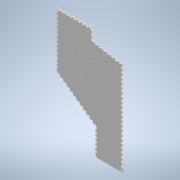
# Autodesk Inventor part: 00_Baseplate_Simmo_base
Saved by Autodesk Inventor 2022 (Build 260153000, 153)
## iProperties
Created: 2022-04-28
Part Number: 00_Baseplate_Simmo_base
Material: Generisch
Document SubType Name: Modeling
Designer: diederichbenedict
Density: 1 g/cm^3
Appearance: Vorgabe
Author: diederichbenedict
Autodesk Inventor part; units mm, degrees
ref_plane "YZ Plane" through (0, 0, 0) normal (1, 0, 0) x (0, 1, 0)
ref_plane "XZ Plane" through (0, 0, 0) normal (0, 1, 0) x (-1, 0, 0)
ref_plane "XY Plane" through (0, 0, 0) normal (0, 0, 1) x (1, 0, 0)
ref_plane "Arbeitsebene1" through (0, 0, 0) normal (0, 0, 1) x (1, 0, 0)
sketch "Skizze1" plane through (0, 0, 0) normal (0, 0, 1) x (1, 0, 0)
  line L0 (91.8818, 443.0401) -> (90.2278, 433.6598) projected
  line L1 (120, 0) -> (126, 0)
  line L2 (126, 0) -> (126, 460)
  line L3 (126, 460) -> (-21.6976, 486.0431)
  line L4 (-21.6976, 538.0431) -> (-196, 538.0431)
  line L5 (-196, 538.0431) -> (-196, 268.0431)
  line L6 (-196, 268.0431) -> (-6, 130)
  line L7 (-6, 130) -> (-6, 0)
  circle A0 centre (58.4, 5) radius 1.4 projected
  line L8 (88.6, 0) -> (31.4, 0) projected
  line L9 (87.5, 10) -> (32.5, 10) projected
  line L10 (120, 0) -> (0, 0)
  line L11 (126, 0) -> (-6, 0)
  line L12 (64.2504, 447.9123) -> (88.7659, 443.5895) construction
  line L13 (-114.6675, 285.8993) -> (-136.5111, 301.7696) construction
  line L14 (-134.4827, 366.1267) -> (-158.3225, 378.8026) construction
  line L15 (-21.6976, 486.0431) -> (-21.6976, 538.0431)
  circle A1 centre (78.4, 5) radius 1.4 projected
  circle A2 centre (38.4, 5) radius 1.4 projected
  circle A3 centre (100.9244, 442.0092) radius 4 construction
  circle A4 centre (31.4122, 427.865) radius 4 construction
  circle A5 centre (96.4095, 416.4042) radius 4 construction
  circle A6 centre (35.927, 453.47) radius 4 construction
  line L16 (51.7328, 440.252) -> (83.0647, 434.7274) construction
  line L17 (83.0647, 434.7274) -> (84.7881, 444.5016) construction
  line L18 (84.7881, 444.5016) -> (53.4563, 450.0262) construction
  line L19 (53.4563, 450.0262) -> (51.7328, 440.252) construction
  line L20 (80.7877, 445.6487) -> (93.6153, 443.3868) construction
  line L21 (93.6153, 443.3868) -> (94.8156, 450.1944) construction
  line L22 (94.8156, 450.1944) -> (106.0791, 448.2083) construction
  arc A7 (108.5126, 444.7329) -> (106.0791, 448.2083) centre (105.5582, 445.2539) ccw construction
  line L23 (108.5126, 444.7329) -> (102.6086, 411.2495) construction
  arc A8 (99.1332, 408.816) -> (102.6086, 411.2495) centre (99.6541, 411.7704) ccw construction
  line L24 (99.1332, 408.816) -> (26.2574, 421.666) construction
  arc A9 (23.8239, 425.1413) -> (26.2574, 421.666) centre (26.7784, 424.6204) ccw construction
  line L25 (23.8239, 425.1413) -> (29.728, 458.6248) construction
  arc A10 (33.2033, 461.0583) -> (29.728, 458.6248) centre (32.6824, 458.1038) ccw construction
  line L26 (33.2033, 461.0583) -> (44.5085, 459.0649) construction
  line L27 (44.5085, 459.0649) -> (43.3082, 452.2573) construction
  line L28 (43.3082, 452.2573) -> (56.1358, 449.9955) construction
  line L29 (56.1358, 449.9955) -> (57.3361, 456.803) construction
  line L30 (57.3361, 456.803) -> (81.988, 452.4562) construction
  line L31 (81.988, 452.4562) -> (80.7877, 445.6487) construction
  line L32 (32.5, 5.1) -> (32.5, 10) projected
  line L33 (87.5, 10) -> (87.5, 5.1) projected
  line L34 (87.5, 5.1) -> (88.6, 5.1) projected
  line L35 (88.6, 5.1) -> (88.6, 0) projected
  line L36 (31.4, 0) -> (31.4, 5.1) projected
  line L37 (31.4, 5.1) -> (32.5, 5.1) projected
  point P0 (126, 5)
  dimension "d1" = 90
  dimension "d66" = 130
  dimension "d69" = 460
  dimension "d70" = 190
  dimension "d71" = 270
  constraints: 20 end point, 3 horizontal, 3 parallel, 1 perpendicular, 1 point on line, 1 vertical
  measures "d1" angle of L5 L4
  measures "d66" vertical distance of L1.start L6.end
  measures "d69" distance of L1.end L2.end
  measures "d70" distance between parallel lines of L5 L7
  measures "d71" distance of L4.end L5.end
extrude "Extrusion1" add sketch "Skizze1" along normal blind 6 contours L10 L35 L34 L33 L9 L32 L37 L36 L11 L7 L6 L5 L4 L15 L3 L2 L1 | L8 L36 L37 L32 L9 L33 L34 L35 | A0 | A1 | A2
sketch "Skizze2" plane through (0, 0, 0) normal (0, 0, -1) x (-1, 0, 0)
  line L0 (-126, 0) -> (-120, 0)
  line L1 (-120, 0) -> (-120, 10)
  line L2 (-120, 10) -> (-126, 10)
  line L3 (-126, 10) -> (-126, 0)
  circle A0 centre (-123, 15) radius 1.5
  point P0 (0, 0)
  dimension "d8" = 6
  dimension "d9" = 10
  dimension "d15" = 3
  dimension "d16" = 5
  constraints: 8 end point, 2 parallel, 2 point on line, 1 centre point, 1 horizontal, 1 perpendicular
  measures "d8" distance of L2.end L1.end
  measures "d9" distance of L1.end L0.end
  measures "d15" diameter of A0
  measures "d16" distance from line of A0.centre L2
extrude "Extrusion2" cut sketch "Skizze2" against normal through all
sketch "Skizze3" plane through (0, 0, 0) normal (0, 0, -1) x (-1, 0, 0)
  line L0 (196, 268.0431) -> (6, 130) projected
  line L1 (196, 538.0431) -> (196, 268.0431) projected
  line L2 (21.6976, 538.0431) -> (196, 538.0431) projected
  line L3 (-126, 460) -> (21.6976, 486.0431) projected
pattern_linear "Rechteckige Anordnung1" count 24 spacing 20 along (0, 1, 0) of "Extrusion2"
sketch "Skizze4" plane through (0, 0, 0) normal (0, 0, -1) x (-1, 0, 0)
  line L0 (-120, 461.058) -> (-110.1519, 462.7944)
  line L1 (-110.1519, 462.7944) -> (-109.11, 456.8856)
  line L2 (-109.11, 456.8856) -> (-118.9581, 455.1491)
  line L3 (-118.9581, 455.1491) -> (-120, 461.058)
  circle A0 centre (-104.7069, 460.7083) radius 1.5
  line L4 (-126, 460) -> (21.6976, 486.0431) projected
  line L5 (-120, 0) -> (-120, 9.8) projected
  point P0 (0, 0)
  dimension "d17" = 10
  dimension "d18" = 6
  dimension "d19" = 3
  dimension "d20" = 5
  dimension "d73" = 3
  constraints: 8 end point, 2 parallel, 2 point on line, 1 centre point, 1 collinear, 1 perpendicular
  measures "d17" distance of L1.end L2.end
  measures "d18" distance of L0.end L1.end
  measures "d19" diameter of A0
  measures "d20" distance from line of A0.centre L1
  measures "d73" distance from line of L2 A0.centre
extrude "Extrusion3" cut sketch "Skizze4" against normal through all
pattern_linear "Rechteckige Anordnung2" count 7 spacing 20 along (-0.9848078, 0.1736482, 0) of "Extrusion3"
sketch "Skizze5" plane through (0, 0, 0) normal (0, 0, -1) x (-1, 0, 0)
  line L0 (21.6976, 538.0431) -> (21.6976, 532.0431)
  line L1 (21.6976, 532.0431) -> (31.6976, 532.0431)
  line L2 (31.6976, 532.0431) -> (31.6976, 538.0431)
  line L3 (31.6976, 538.0431) -> (21.6976, 538.0431)
  circle A0 centre (36.6976, 535.0431) radius 1.5
  line L4 (21.6976, 538.0431) -> (196, 538.0431) projected
  point P0 (0, 0)
  dimension "d29" = 6
  dimension "d30" = 10
  dimension "d31" = 3
  dimension "d32" = 5
  constraints: 8 end point, 2 parallel, 1 centre point, 1 coincident, 1 collinear, 1 perpendicular
  measures "d29" distance of L0.start L0.end
  measures "d30" distance of L1.end L0.end
  measures "d31" diameter of A0
  measures "d32" distance from line of A0.centre L2
extrude "Extrusion4" cut sketch "Skizze5" against normal through all
pattern_linear "Rechteckige Anordnung3" count 9 spacing 20 along (-1, 0, 0) of "Extrusion4"
sketch "Skizze6" plane through (0, 0, 0) normal (0, 0, -1) x (-1, 0, 0)
  line L0 (196, 538.0431) -> (196, 268.0431) projected
  line L1 (196, 532.0431) -> (190, 532.0431)
  line L2 (190, 532.0431) -> (190, 522.0431)
  line L3 (190, 522.0431) -> (196, 522.0431)
  line L4 (196, 522.0431) -> (196, 532.0431)
  circle A0 centre (193, 517.0431) radius 1.5
  line L5 (31.6976, 538.0431) -> (196, 538.0431) projected
  point P0 (0, 0)
  point P1 (196, 344.793)
  point P2 (196, 522.0431)
  point P3 (191.6976, 538.0431)
  dimension "d38" = 6
  dimension "d39" = 10
  dimension "d40" = 3
  dimension "d41" = 5
  dimension "d74" = 6
  dimension "d75" = 3
  constraints: 6 end point, 2 horizontal, 1 centre point, 1 parallel, 1 point on line, 1 vertical, 3 other
  measures "d38" distance of L1.start L1.end
  measures "d39" distance of L3.start L1.end
  measures "d40" diameter of A0
  measures "d41" distance from line of A0.centre L3
  measures "d74" distance between parallel lines of L1 L5
  measures "d75" distance from line of A0.centre L4
extrude "Extrusion5" cut sketch "Skizze6" against normal through all
pattern_linear "Rechteckige Anordnung4" count 24 spacing 20 along (0, -1, 0) of "Extrusion5"
sketch "Skizze7" plane through (0, 0, 0) normal (0, 0, -1) x (-1, 0, 0)
  line L0 (196, 268.0431) -> (6, 130) projected
  line L1 (196, 268.0431) -> (6, 130) projected
  line L2 (189.8762, 263.5939) -> (186.3495, 268.448)
  line L3 (186.3495, 268.448) -> (178.2593, 262.5701)
  line L4 (178.2593, 262.5701) -> (181.7861, 257.716)
  line L5 (181.7861, 257.716) -> (189.8762, 263.5939)
  line L6 (189.8762, 263.5939) -> (195.8762, 263.5939) construction
  circle A0 centre (175.9776, 257.2042) radius 1.5
  point P0 (0, 0)
  point P1 (181.7861, 257.716)
  point P2 (192.6247, 295.5908)
  point P3 (185.8311, 260.655)
  point P4 (190, 302.0431)
  dimension "d47" = 6
  dimension "d49" = 10
  dimension "d50" = 3
  dimension "d51" = 5
  dimension "d76" = 3
  dimension "d77" = 22.7
  constraints: 10 end point, 2 parallel, 2 perpendicular, 1 centre point, 1 equal length, 1 horizontal, 1 midpoint, 2 other
  measures "d47" distance of L2.start L2.end
  measures "d49" distance of L3.end L2.end
  measures "d50" diameter of A0
  measures "d51" distance from line of L4 A0.centre
  measures "d76" distance from line of A0.centre L5
  measures "d77" distance from line of point (190, 302.043) L2
extrude "Extrusion6" cut sketch "Skizze7" against normal through all
pattern_linear "Rechteckige Anordnung5" count 12 spacing 20 along (0.809017, -0.5877853, 0) of "Extrusion6"
sketch "Skizze8" plane through (0, 0, 0) normal (0, 0, -1) x (-1, 0, 0)
  circle A0 centre (3, 15) radius 1.5
  line L0 (6, 130) -> (6, 0) projected
  line L1 (6, 0) -> (0, 0)
  line L2 (0, 0) -> (0, 10)
  line L3 (0, 10) -> (6, 10)
  line L4 (6, 10) -> (6, 0)
  dimension "d94" = 6
  dimension "d95" = 10
  dimension "d96" = 5
  constraints: 8 end point, 2 parallel, 1 centre point, 1 horizontal, 1 perpendicular
  measures "d94" distance of L2.end L3.end
  measures "d95" distance of L1.end L2.end
  measures "d96" distance from line of A0.centre L3
extrude "Extrusion7" cut sketch "Skizze8" against normal through all
pattern_linear "Rechteckige Anordnung6" count 6 spacing 20 along (0, 1, 0) of "Extrusion7"
sketch "Skizze9" plane through (0, 0, 0) normal (0, 0, -1) x (-1, 0, 0)
  circle A0 centre (75.7794, 274.2099) radius 4 projected
  circle A1 centre (5.0617, 279.7773) radius 4 projected
  circle A2 centre (68.1778, 299.0739) radius 4 projected
  circle A3 centre (12.6633, 254.9134) radius 4 projected
  line L0 (26.7404, 269.9591) -> (57.1654, 279.261) projected
  line L1 (57.1654, 279.261) -> (60.0672, 269.7697) projected
  line L2 (60.0672, 269.7697) -> (29.6422, 260.4678) projected
  line L3 (29.6422, 260.4678) -> (26.7404, 269.9591) projected
  line L4 (56.2364, 268.1436) -> (68.6927, 271.9519) projected
  line L5 (68.6927, 271.9519) -> (70.7137, 265.3414) projected
  line L6 (70.7137, 265.3414) -> (81.6513, 268.6853) projected
  arc A4 (81.6513, 268.6853) -> (83.6431, 272.4313) centre (80.7741, 271.5542) ccw projected
  line L7 (83.6431, 272.4313) -> (73.7024, 304.9457) projected
  arc A5 (73.7024, 304.9457) -> (69.9564, 306.9375) centre (70.8335, 304.0686) ccw projected
  line L8 (69.9564, 306.9375) -> (-0.8102, 285.302) projected
  arc A6 (-0.8102, 285.302) -> (-2.802, 281.556) centre (0.067, 282.4331) ccw projected
  line L9 (-2.802, 281.556) -> (7.1387, 249.0416) projected
  arc A7 (7.1387, 249.0416) -> (10.8847, 247.0498) centre (10.0076, 249.9187) ccw projected
  line L10 (10.8847, 247.0498) -> (21.8627, 250.4061) projected
  line L11 (21.8627, 250.4061) -> (19.8417, 257.0166) projected
  line L12 (19.8417, 257.0166) -> (32.298, 260.8249) projected
  line L13 (32.298, 260.8249) -> (34.319, 254.2144) projected
  line L14 (34.319, 254.2144) -> (58.2574, 261.5331) projected
  line L15 (58.2574, 261.5331) -> (56.2364, 268.1436) projected
  line L16 (59.7195, 410.0053) -> (29.1368, 401.2359) projected
  line L17 (29.1368, 401.2359) -> (26.4011, 410.7764) projected
  line L18 (26.4011, 410.7764) -> (56.9838, 419.5459) projected
  line L19 (56.9838, 419.5459) -> (59.7195, 410.0053) projected
  line L20 (30.2597, 412.3354) -> (17.7388, 408.7451) projected
  line L21 (17.7388, 408.7451) -> (15.8334, 415.3898) projected
  line L22 (15.8334, 415.3898) -> (4.8392, 412.2373) projected
  line L23 (2.7824, 408.5266) -> (12.154, 375.8437) projected
  line L24 (15.8647, 373.7868) -> (86.9981, 394.184) projected
  line L25 (89.055, 397.8947) -> (79.6833, 430.5776) projected
  line L26 (75.9726, 432.6345) -> (64.9377, 429.4703) projected
  line L27 (64.9377, 429.4703) -> (66.8431, 422.8255) projected
  line L28 (66.8431, 422.8255) -> (54.3222, 419.2352) projected
  line L29 (54.3222, 419.2352) -> (52.4168, 425.88) projected
  line L30 (52.4168, 425.88) -> (28.3543, 418.9801) projected
  line L31 (28.3543, 418.9801) -> (30.2597, 412.3354) projected
  circle A8 centre (-100.9244, 442.0092) radius 4 projected
  circle A9 centre (-31.4122, 427.865) radius 4 projected
  circle A10 centre (-96.4095, 416.4042) radius 4 projected
  circle A11 centre (-35.927, 453.47) radius 4 projected
  line L32 (-51.7328, 440.252) -> (-83.0647, 434.7274) projected
  line L33 (-83.0647, 434.7274) -> (-84.7881, 444.5016) projected
  line L34 (-84.7881, 444.5016) -> (-53.4563, 450.0262) projected
  line L35 (-53.4563, 450.0262) -> (-51.7328, 440.252) projected
  line L36 (-80.7877, 445.6487) -> (-93.6153, 443.3868) projected
  line L37 (-93.6153, 443.3868) -> (-94.8156, 450.1944) projected
  line L38 (-94.8156, 450.1944) -> (-106.0791, 448.2083) projected
  arc A12 (-106.0791, 448.2083) -> (-108.5126, 444.7329) centre (-105.5582, 445.2539) ccw projected
  line L39 (-108.5126, 444.7329) -> (-102.6086, 411.2495) projected
  arc A13 (-102.6086, 411.2495) -> (-99.1332, 408.816) centre (-99.6541, 411.7704) ccw projected
  line L40 (-99.1332, 408.816) -> (-26.2574, 421.666) projected
  arc A14 (-26.2574, 421.666) -> (-23.8239, 425.1413) centre (-26.7784, 424.6204) ccw projected
  line L41 (-23.8239, 425.1413) -> (-29.728, 458.6248) projected
  arc A15 (-29.728, 458.6248) -> (-33.2033, 461.0583) centre (-32.6824, 458.1038) ccw projected
  line L42 (-33.2033, 461.0583) -> (-44.5085, 459.0649) projected
  line L43 (-44.5085, 459.0649) -> (-43.3082, 452.2573) projected
  line L44 (-43.3082, 452.2573) -> (-56.1358, 449.9955) projected
  line L45 (-56.1358, 449.9955) -> (-57.3361, 456.803) projected
  line L46 (-57.3361, 456.803) -> (-81.988, 452.4562) projected
  line L47 (-81.988, 452.4562) -> (-80.7877, 445.6487) projected
  circle A16 centre (40.3846, 517.8974) radius 4 projected
  circle A17 centre (109.8967, 503.7532) radius 4 projected
  circle A18 centre (44.8994, 492.2924) radius 4 projected
  circle A19 centre (105.3819, 529.3582) radius 4 projected
  line L48 (89.5761, 516.1402) -> (58.2443, 510.6156) projected
  line L49 (58.2443, 510.6156) -> (56.5208, 520.3898) projected
  line L50 (56.5208, 520.3898) -> (87.8527, 525.9145) projected
  line L51 (87.8527, 525.9145) -> (89.5761, 516.1402) projected
  line L52 (60.5212, 521.5369) -> (47.6937, 519.275) projected
  line L53 (47.6937, 519.275) -> (46.4933, 526.0826) projected
  line L54 (46.4933, 526.0826) -> (35.2298, 524.0965) projected
  arc A20 (35.2298, 524.0965) -> (32.7963, 520.6211) centre (35.7507, 521.1421) ccw projected
  line L55 (32.7963, 520.6211) -> (38.7004, 487.1377) projected
  arc A21 (38.7004, 487.1377) -> (42.1757, 484.7042) centre (41.6548, 487.6586) ccw projected
  line L56 (42.1757, 484.7042) -> (115.0515, 497.5542) projected
  arc A22 (115.0515, 497.5542) -> (117.485, 501.0295) centre (114.5306, 500.5086) ccw projected
  line L57 (117.485, 501.0295) -> (111.5809, 534.513) projected
  arc A23 (111.5809, 534.513) -> (108.1056, 536.9465) centre (108.6265, 533.992) ccw projected
  line L58 (108.1056, 536.9465) -> (96.8004, 534.9531) projected
  line L59 (96.8004, 534.9531) -> (98.0007, 528.1455) projected
  line L60 (98.0007, 528.1455) -> (85.1732, 525.8837) projected
  line L61 (85.1732, 525.8837) -> (83.9728, 532.6912) projected
  line L62 (83.9728, 532.6912) -> (59.3209, 528.3444) projected
  line L63 (59.3209, 528.3444) -> (60.5212, 521.5369) projected
  circle A24 centre (10.6137, 406.611) radius 4 projected
  circle A25 centre (81.2236, 399.8103) radius 4 projected
  circle A26 centre (17.7803, 381.6182) radius 4 projected
  circle A27 centre (74.057, 424.8031) radius 4 projected
  arc A28 (4.8392, 412.2373) -> (2.7824, 408.5266) centre (5.6661, 409.3535) ccw projected
  arc A29 (12.154, 375.8437) -> (15.8647, 373.7868) centre (15.0378, 376.6706) ccw projected
  arc A30 (86.9981, 394.184) -> (89.055, 397.8947) centre (86.1712, 397.0678) ccw projected
  arc A31 (79.6833, 430.5776) -> (75.9726, 432.6345) centre (76.7995, 429.7507) ccw projected
  point P0 (0, 0)
hole "Bohrung1" at (-12.6633, 254.9134, 0) at (-5.0617, 279.7773, 0) at (-75.7794, 274.2099, 0) at (-68.1778, 299.0739, 0) at (-44.8994, 492.2924, 0) at (-40.3846, 517.8974, 0) at (-109.8967, 503.7532, 0) at (-105.3819, 529.3582, 0) at (31.4122, 427.865, 0) at (35.927, 453.47, 0) at (96.4095, 416.4042, 0) at (100.9244, 442.0092, 0) at (-17.7803, 381.6182, 0) at (-81.2236, 399.8103, 0) at (-74.057, 424.8031, 0) at (-10.6137, 406.611, 0) direction (0, 0, 1) diameter 2.8 depth 8 tip angle 118
sketch "Skizze10" plane through (0, 0, 0) normal (0, 0, -1) x (-1, 0, 0)
  line L0 (21.6976, 486.0431) -> (21.6976, 532.0431) projected
  line L1 (21.6976, 486.0431) -> (27.6976, 486.0431)
  line L2 (27.6976, 486.0431) -> (27.6976, 496.0431)
  line L3 (27.6976, 496.0431) -> (21.6976, 496.0431)
  line L4 (21.6976, 496.0431) -> (21.6976, 486.0431)
  circle A0 centre (24.6976, 501.0431) radius 1.5
  point P0 (0, 0)
  dimension "d85" = 6
  dimension "d86" = 10
  dimension "d87" = 3
  dimension "d88" = 5
  constraints: 8 end point, 2 parallel, 1 centre point, 1 horizontal, 1 perpendicular
  measures "d85" distance of L3.end L2.end
  measures "d86" distance of L2.end L1.end
  measures "d87" diameter of A0
  measures "d88" distance from line of A0.centre L3
extrude "Extrusion8" cut sketch "Skizze10" against normal blind 10
pattern_linear "Rechteckige Anordnung7" count 3 spacing 20 along (0, 1, 0) of "Extrusion8"
equation "\"d16\" = 0.5 * d9"
equation "\"d17\" = d9"
equation "\"d20\" = 0.5 * d9"
equation "\"d73\" = 0.5 * d18"
equation "\"d25\" = 2 * d9"
equation "\"d30\" = d9"
equation "\"d32\" = 0.5 * d9"
equation "\"d37\" = 2 * d9"
equation "\"d39\" = d9"
equation "\"d41\" = 0.5 * d9"
equation "\"d74\" = d18"
equation "\"d49\" = d9"
equation "\"d51\" = 0.5 * d9"
equation "\"d56\" = 2 * d9"
equation "\"d65\" = 2 * d9"
equation "\"d14\" = 2 * d9"
equation "\"d46\" = 2 * d9"
